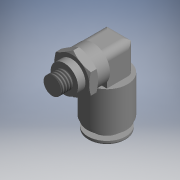
# Autodesk Inventor part: GWJL6-M5
Saved by Autodesk Inventor 2017.3 (Build 213256000, 256)
## iProperties
Part Number: GWJL6-M5
Material: Generic
Catalog Web Link: www.cadenas.de
Description: GWJL*-*-Single elbow
Vendor: CKDCN
Document SubType Name: Modeling
Designer: partserver
Manufacturer: CKDCN
Mass: 7 g
Surface Area: 16.3422 cm^2
Volume: 2.13734 cm^3
Density: 1 g/cm^3
Appearance: PSOLRGB-175-175-175
Category: PARTsolutions
Company: CKDCN
Title: GWJL6-M5
Author: Cadenas PARTsolutions
Comments: Single elbow
PSOL_IDENT_0: {$CADENAS_DATA\23d-libs\ckd_cn\speed_control_check_valves_auxiliary_components\fitting_tube\fitting_
PSOL_IDENT_1: gwj_mini_series\gwjl.prj},158 {VTYP=3D},{NB=GWJL6-M5},{LINA=GWJL6-M5},{NN=GWJL*-*},{DATE=07.08.2020
PSOL_IDENT_2: 12:08:08},{GEOMDATE=21.07.2020 09:34:03},{VERSION=},{LINEID=140},{WBVAR=},{WBNUMERIC=}  {NB=GWJL6-M5
PSOL_IDENT_3: },{LINA=GWJL6-M5},{KT=DUMMY},{IDNR=},{MODEL=GWJL6-M5},{BORE=6.0},{THREAD=M5x0.8},{NDM=5.000},{P=0.80
PSOL_IDENT_4: 0},{HEX=10},{L1=15.5},{L2=18.5},{A=3.4},{B=14.5},{C=11.8},{MBS=2.5},{ESA=3.5},{WEIGHT=7.0},{INFOTEXT=
PSOL_IDENT_5: Dimensions},{CNSORDERNO=GWJL6-M5}
NB: GWJL6-M5
NN: GWJL*-*
NT: Single elbow
NBSYN: $MODEL.
LINA: GWJL6-M5
CATALOG: CKD
MODEL: GWJL6-M5
BORE: 6
THREAD: M5x0.8
HEX: 10
L1: 15.5
L2: 18.5
A: 3.4
B: 14.5
C: 11.8
MBS: 2.5
ESA: 3.5
WEIGHT: 7
INFOTEXT: Dimensions
SUPPLIER: CKDCN
ARTICLENO: GWJL6-M5
BOMINFO: GWJL6-M5
CREATOR: CADENAS GmbH
Autodesk Inventor part; units mm, degrees
ref_plane "YZ Plane" through (0, 0, 0) normal (1, 0, 0) x (0, 1, 0)
ref_plane "XZ Plane" through (0, 0, 0) normal (0, 1, 0) x (-1, 0, 0)
ref_plane "XY Plane" through (0, 0, 0) normal (0, 0, 1) x (1, 0, 0)
sketch "Sketch_20" plane through (0, 0, 0) normal (1, 0, 0) x (0, 1, 0)
  line L0 (19.5, -14.1) -> (11.5, -14.1)
  line L1 (11.5, -14.1) -> (11.5, -22.5)
  line L2 (11.5, -22.5) -> (17.5, -22.5)
  arc A0 (17.5, -22.5) -> (19.5, -20.5) centre (17.5, -20.5) ccw
  line L3 (19.5, -20.5) -> (19.5, -14.1)
  constraints: 8 end point, 2 point on circle, 1 centre point
extrude "Extrusion1" add sketch "Sketch_20" along normal mid plane 8
sketch "Sketch_2" plane through (0, 0, 0) normal (0, 0, 1) x (1, 0, 0)
  line L0 (-10, 5) -> (10, 5)
  line L1 (10, 5) -> (10, 25)
  line L2 (10, 25) -> (-10, 25)
  line L3 (-10, 25) -> (-10, 5)
  line L4 (-4, 11.5) -> (4, 11.5)
  line L5 (4, 11.5) -> (4, 17.5)
  arc A0 (4, 17.5) -> (2, 19.5) centre (2, 17.5) ccw
  line L6 (2, 19.5) -> (-2, 19.5)
  arc A1 (-2, 19.5) -> (-4, 17.5) centre (-2, 17.5) ccw
  line L7 (-4, 17.5) -> (-4, 11.5)
  constraints: 16 end point, 4 point on circle, 2 centre point
extrude "Extrusion2" cut sketch "Sketch_2" along normal mid plane 57
sketch "Sketch_13" plane through (0, 0, 0) normal (0, 1, 0) x (-1, 0, 0)
  line L0 (10, -10) -> (-10, -10)
  line L1 (-10, -10) -> (-10, -25)
  line L2 (-10, -25) -> (10, -25)
  line L3 (10, -25) -> (10, -10)
  line L4 (4, -20.5) -> (4, -12.5)
  line L5 (4, -12.5) -> (-4, -12.5)
  line L6 (-4, -12.5) -> (-4, -20.5)
  arc A0 (-4, -20.5) -> (-2, -22.5) centre (-2, -20.5) ccw
  line L7 (-2, -22.5) -> (2, -22.5)
  arc A1 (2, -22.5) -> (4, -20.5) centre (2, -20.5) ccw
  constraints: 16 end point, 4 point on circle, 2 centre point
extrude "Extrusion3" cut sketch "Sketch_13" along normal blind 25
sketch "Sketch_12" plane through (0, 0, 0) normal (1, 0, 0) x (0, 1, 0)
  line L0 (3.4, -18.5) -> (11.5, -18.5)
  line L1 (11.5, -18.5) -> (11.5, -23.4)
  line L2 (11.5, -23.4) -> (8, -23.4)
  line L3 (8, -23.4) -> (8, -23.5)
  line L4 (8, -23.5) -> (7.4226, -24.5)
  line L5 (7.4226, -24.5) -> (6.0774, -24.5)
  line L6 (6.0774, -24.5) -> (5.5, -23.5)
  line L7 (5.5, -23.5) -> (5.5, -22.4)
  line L8 (5.5, -22.4) -> (3.4, -22.4)
  line L9 (3.4, -22.4) -> (3.4, -18.5)
  line L10 (3.4, -18.5) -> (11.5, -18.5)
  constraints: 22 end point
revolve "Revolution1" add sketch "Sketch_12" angle 360 about axis through (0, 3.4, -18.5) along (0, -1, 0)
sketch "Sketch_6" plane through (0, 0, 0) normal (0, 1, 0) x (-1, 0, 0)
  line L0 (10, -8.5) -> (-10, -8.5)
  line L1 (-10, -8.5) -> (-10, -28.5)
  line L2 (-10, -28.5) -> (10, -28.5)
  line L3 (10, -28.5) -> (10, -8.5)
  line L4 (5, -15.6132) -> (0, -12.7265)
  line L5 (0, -12.7265) -> (-5, -15.6132)
  line L6 (-5, -15.6132) -> (-5, -21.3868)
  line L7 (-5, -21.3868) -> (0, -24.2735)
  line L8 (0, -24.2735) -> (5, -21.3868)
  line L9 (5, -21.3868) -> (5, -15.6132)
  constraints: 20 end point
extrude "Extrusion4" cut sketch "Sketch_6" along normal blind 10
sketch "Sketch_7" plane through (0, 0, 0) normal (1, 0, 0) x (0, 1, 0)
  line L0 (0, -18.5) -> (3.4, -18.5)
  line L1 (3.4, -18.5) -> (3.4, -21)
  line L2 (3.4, -21) -> (0, -21)
  line L3 (0, -21) -> (0, -18.5)
  line L4 (0, -18.5) -> (3.4, -18.5)
  constraints: 10 end point
revolve "Revolution2" add sketch "Sketch_7" angle 360 about axis through (0, 0, -18.5) along (0, -1, 0)
thread "Thread1" size "M5x0.8" class "6g" standard "ISO Metric profile" full length
sketch "Sketch_15" plane through (0, 0, 0) normal (1, 0, 0) x (0, 1, 0)
  line L0 (15.5, -14.1) -> (15.5, 0)
  line L1 (15.5, 0) -> (20.4, 0)
  arc A0 (20.9, -0.5) -> (20.4, 0) centre (20.4, -0.5) ccw
  line L2 (20.9, -0.5) -> (20.9, -1)
  line L3 (20.9, -1) -> (19.1, -1)
  line L4 (19.1, -1) -> (19.1, -2.6)
  line L5 (19.1, -2.6) -> (21, -2.6)
  line L6 (21, -2.6) -> (21, -3.6)
  line L7 (21, -3.6) -> (21.4, -3.6)
  line L8 (21.4, -3.6) -> (21.4, -14.1)
  line L9 (21.4, -14.1) -> (15.5, -14.1)
  line L10 (15.5, -14.1) -> (15.5, 0)
  constraints: 22 end point, 2 point on circle, 1 centre point
revolve "Revolution3" add sketch "Sketch_15" angle 360 about axis through (0, 15.5, -14.1) along (0, 0, -1)
sketch "Sketch_18" plane through (0, 0, 0) normal (1, 0, 0) x (0, 1, 0)
  line L0 (15.5, -14.5) -> (15.5, 0)
  line L1 (15.5, 0) -> (18.5, 0)
  line L2 (18.5, 0) -> (18.5, -14.5)
  line L3 (18.5, -14.5) -> (15.5, -14.5)
  line L4 (15.5, -14.5) -> (15.5, 0)
  constraints: 10 end point
revolve "Revolution4" cut sketch "Sketch_18" angle 360 about axis through (0, 15.5, -14.5) along (0, 0, -1)
body "Solid1"
